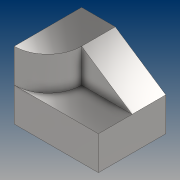
# Autodesk Inventor part: 39
Saved by Autodesk Inventor 2020.2 (Build 242310000, 310)
## iProperties
Created: 2020-09-17
Part Number: 39
Material: 鋼、碳鋼
Document SubType Name: Modeling
Designer: user
Density: 7.85 g/cm^3
Appearance: 半拋光
Mass: 473.223 g
Surface Area: 101.494 cm^2
Volume: 60.2832 cm^3
Author: user
Autodesk Inventor part; units mm, degrees
ref_plane "YZ Plane" through (0, 0, 0) normal (1, 0, 0) x (0, 1, 0)
ref_plane "XZ Plane" through (0, 0, 0) normal (0, 1, 0) x (-1, 0, 0)
ref_plane "XY Plane" through (0, 0, 0) normal (0, 0, 1) x (1, 0, 0)
sketch "草圖1" plane through (0, 0, 0) normal (0, 1, 0) x (-1, 0, 0)
  line L0 (0, 0) -> (-50, 0)
  line L1 (-50, 0) -> (-50, 40)
  line L2 (-50, 40) -> (0, 40)
  line L3 (0, 40) -> (0, 0)
  dimension "d0" = 50
  dimension "d1" = 40
  constraints: 8 end point, 2 parallel, 1 horizontal, 1 perpendicular
  measures "d0" distance of L1.end L2.end
  measures "d1" distance of L2.end L0.start
extrude "擠出1" add sketch "草圖1" along normal blind 40
sketch "草圖2" plane through (0, 0, 40) normal (0, 0, 1) x (1, 0, 0)
  line L0 (0, 0) -> (0, 40) projected
  line L1 (0, 40) -> (50, 40) projected
  line L2 (50, 40) -> (50, 0) projected
  line L3 (50, 0) -> (0, 0) projected
  line L4 (50, 20) -> (20, 40)
  line L5 (50, 0) -> (50, 40) projected
  point P0 (50, 20)
  dimension "d4" = 30
  dimension "d5" = 20
  constraints: 2 end point, 1 midpoint, 1 point on line
  measures "d4" distance from line of L2 L4.end
  measures "d5" distance from line of L1 L4.start
extrude "擠出2" cut sketch "草圖2" against normal through all contours L1 L2 L4
sketch "草圖3" plane through (0, 40, 0) normal (0, 1, 0) x (1, 0, 0)
  line L0 (20, 0) -> (20, -40) projected
  line L1 (20, -40) -> (0, -40) projected
  line L2 (0, -40) -> (0, 0) projected
  line L3 (0, 0) -> (20, 0) projected
  line L4 (20, -20) -> (50, -20)
  line L5 (50, -20) -> (50, -40)
  line L6 (50, -40) -> (20, -40)
  line L7 (20, -40) -> (20, -20)
  line L8 (0, -40) -> (20, -40) projected
  line L9 (50, 0) -> (50, -40) projected
  dimension "d8" = 20
  constraints: 8 end point, 3 collinear, 2 parallel, 1 horizontal, 1 perpendicular
  measures "d8" distance between parallel lines of L4 L6
extrude "擠出3" cut sketch "草圖3" against normal up to surface (20 mm away) contours L4 L5 L6 L0
fillet "圓角1" radius 20 1 edges at (20, 30, 40)
